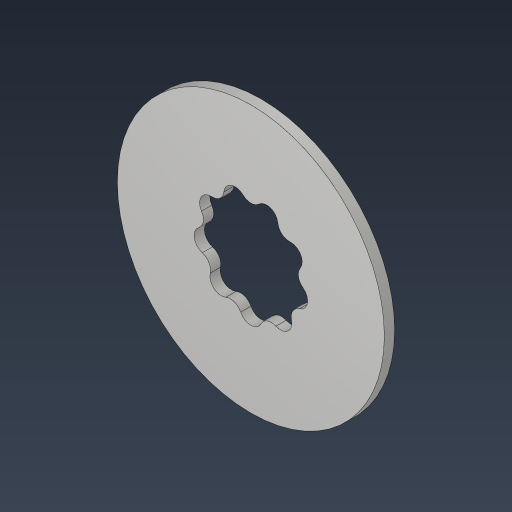
# Autodesk Inventor part: Encoder Disk Halter
Saved by Autodesk Inventor 2023.1 (Build 271208000, 208)
## iProperties
Part Number: Encoder Disk Halter
Material: Aluminium 6061
Document SubType Name: Modeling
Designer: rYan
Mass: 1.93169 g
Surface Area: 12.7104 cm^2
Volume: 0.71544 cm^3
Density: 2.7 g/cm^3
Appearance: Aluminium - flach
Author: rYan
Autodesk Inventor part; units mm, degrees
ref_plane "YZ Plane" through (0, 0, 0) normal (1, 0, 0) x (0, 1, 0)
ref_plane "XZ Plane" through (0, 0, 0) normal (0, 1, 0) x (-1, 0, 0)
ref_plane "XY Plane" through (0, 0, 0) normal (0, 0, 1) x (1, 0, 0)
sketch "Skizze1" plane through (0, 0, 0) normal (1, 0, 0) x (0, 1, 0)
  line L0 (0, 0) -> (5, 0)
  line L1 (0, 5.6) -> (0, 13)
  line L2 (0, 13) -> (1, 13)
  line L3 (1, 13) -> (1, 5.6)
  line L4 (0, 5.6) -> (1, 5.6)
  dimension "d0" = 1
  dimension "d1" = 26
  dimension "d55" = 11.2
  constraints: 10 end point, 2 horizontal, 2 perpendicular, 1 point on line
  measures "d0" distance of L1.end L2.end
  measures "d1" diameter of L2 L0
  measures "d55" diameter of L4 L0
revolve "Umdrehung1" add sketch "Skizze1" angle 360 about axis through (0, 0, 0) along (0, 1, 0)
sketch "Skizze7" plane through (0, 0, 0) normal (0, 1, 0) x (-1, 0, 0)
  circle A0 centre (0, 0) radius 5.6
  line L0 (0, 0) -> (0, 5.6) construction
  line L1 (0, 0) -> (3.599611, 4.289849) construction
  arc A1 (-0.769545, 5.014619) -> (-1.915313, 5.262279) centre (-1.539091, 4.228617) ccw
  arc A2 (1.915313, 5.262279) -> (0.769545, 5.014619) centre (1.539091, 4.228617) ccw
  arc A3 (-0.769545, 5.014619) -> (0.769545, 5.014619) centre (0, 5.800622) ccw
  line L2 (1.915313, 5.262279) -> (0, 0) construction
  point P0 (0, 0)
  point P1 (0, 4.700622)
  dimension "d75" = 40
  dimension "d76" = 1.1
  dimension "d85" = 1.1
  dimension "d86" = 4.70062
  dimension "d87" = 20
  constraints: 11 point on circle, 6 end point, 4 tangent, 3 centre point, 1 vertical, 1 other
  measures "d75" angle of L0 L1
  measures "d76" radius of A1
  measures "d85" radius of A3
  measures "d86" distance of point (0, 0) point (0, 4.701)
  measures "d87" angle of L0 L2
sketch "Skizze7 outline for Extrusion2" plane through (0, 0, 0) normal (0, 1, 0) x (-1, 0, 0)
  arc A0 (-0.769545, 5.014619) -> (0.769545, 5.014619) centre (0, 5.800622) ccw
  arc A1 (-1.915313, 5.262279) -> (-0.769545, 5.014619) centre (-1.539091, 4.228617) cw
  arc A2 (1.915313, 5.262279) -> (-1.915313, 5.262279) centre (0, 0) ccw
  arc A3 (0.769545, 5.014619) -> (1.915313, 5.262279) centre (1.539091, 4.228617) cw
extrude "Extrusion2" add sketch "Skizze7 outline for Extrusion2" along normal up to surface (1 mm away)
pattern_circular "Runde Anordnung1" count 9 over 360 about axis through (0, -10, 0) along (0, 1, 0) of "Extrusion2"
